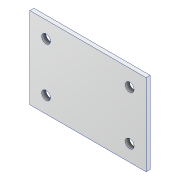
# Autodesk Inventor part: Soporta Potenciómetro
Saved by Autodesk Inventor 2020 (Build 240168000, 168)
## iProperties
Created: 2020-09-22
Part Number: Soporta Potenciómetro
Material: Aluminum 6061
Document SubType Name: Modeling
Designer: Hernan
Density: 2.7 g/cm^3
Appearance: Aluminum - Flat
Author: Hernan
Autodesk Inventor part; units mm, degrees
ref_plane "YZ Plane" through (0, 0, 0) normal (1, 0, 0) x (0, 1, 0)
ref_plane "XZ Plane" through (0, 0, 0) normal (0, 1, 0) x (-1, 0, 0)
ref_plane "XY Plane" through (0, 0, 0) normal (0, 0, 1) x (1, 0, 0)
sketch "Sketch1" plane through (0, 0, 0) normal (0, 0, 1) x (1, 0, 0)
  line L0 (-4.8673, 47.8112) -> (-4.8673, 7.8112)
  line L1 (-4.8673, 7.8112) -> (-61.8673, 7.8112)
  line L2 (-61.8673, 7.8112) -> (-61.8673, 47.8112)
  line L3 (-61.8673, 47.8112) -> (-4.8673, 47.8112)
  circle A0 centre (-53.8673, 15.8112) radius 2.125
  circle A1 centre (-12.8673, 15.8112) radius 2.125
  circle A2 centre (-12.8673, 39.8112) radius 2.125
  circle A3 centre (-53.8673, 39.8112) radius 2.125
  point P0 (0, 0)
  dimension "d0" = 57
  dimension "d1" = 40
  dimension "d18" = 40
  dimension "d20" = 4.25
  dimension "d21" = 4.25
  dimension "d22" = 4.25
  dimension "d23" = 8
  dimension "d25" = 8
  dimension "d26" = 8
  dimension "d27" = 8
  dimension "d28" = 8
  dimension "d29" = 8
  dimension "d30" = 8
  dimension "d31" = 8
  constraints: 8 end point, 4 centre point, 1 parallel
  measures "d0" distance of L0.end L1.end
  measures "d1" distance of L0.start L0.end
  measures "d18" distance of L1.end L2.end
  measures "d20" diameter of A1
  measures "d21" diameter of A2
  measures "d22" diameter of A3
  measures "d23" distance from line of A0.centre L1
  measures "d25" distance from line of L2 A0.centre
  measures "d26" distance from line of A3.centre L2
  measures "d27" distance from line of L3 A3.centre
  measures "d28" distance from line of L0 A2.centre
  measures "d29" distance from line of L3 A2.centre
  measures "d30" distance from line of L0 A1.centre
  measures "d31" distance from line of A1.centre L1
extrude "Extrusion1" add sketch "Sketch1" along normal blind 2
body "Solid1"
